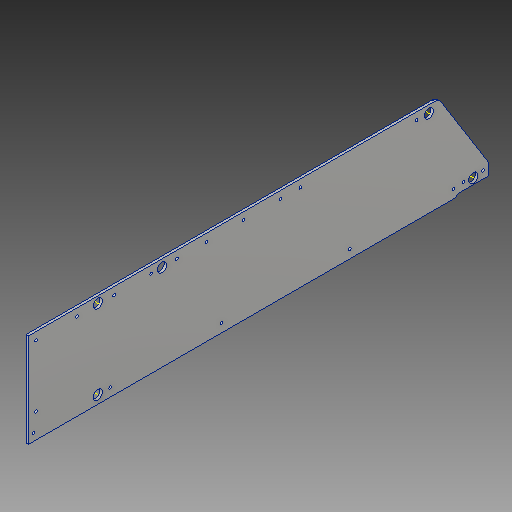
# Autodesk Inventor part: Storage Side Plate
Saved by Autodesk Inventor 2019.4 (Build 234330000, 330)
## iProperties
Created: 2020-01-24
Part Number: Storage Side Plate
Material: Aluminum 6061
Document SubType Name: Modeling
Designer: admin
Density: 2.7 g/cm^3
Appearance: Aluminum - Flat
Mass: 2248.08 g
Surface Area: 3469.21 cm^2
Volume: 832.621 cm^3
Author: admin
Autodesk Inventor part; units mm, degrees
ref_plane "YZ Plane" through (0, 0, 0) normal (1, 0, 0) x (0, 1, 0)
ref_plane "XZ Plane" through (0, 0, 0) normal (0, 1, 0) x (-1, 0, 0)
ref_plane "XY Plane" through (0, 0, 0) normal (0, 0, 1) x (1, 0, 0)
sketch "Sketch1" plane through (0, 0, 0) normal (1, 0, 0) x (0, 1, 0)
  line L0 (0, 0) -> (190, 0)
  line L1 (190, 0) -> (190, -830)
  line L2 (0, -930) -> (0, 0)
  circle A0 centre (95, -413.3735) radius 88.9 construction
  circle A1 centre (177, -140) radius 9.5
  circle A2 centre (17, -140) radius 9.5
  circle A3 centre (17, -900) radius 9.5
  circle A4 centre (175, -810) radius 9.5
  line L3 (17, -140) -> (17, -900) construction
  line L4 (234.971, -205) -> (-89.3496, -205) construction
  circle A5 centre (175, -270) radius 9.5
  line L5 (175, -270) -> (175, -810) construction
  line L6 (17, -140) -> (177, -140) construction
  circle A6 centre (97.3586, -237.1878) radius 88.9 construction
  circle A7 centre (99.6878, -594.5711) radius 88.9 construction
  circle A8 centre (95, -787.6266) radius 88.9 construction
  circle A9 centre (175, -300) radius 2.75
  circle A10 centre (175, -550) radius 2.75
  circle A11 centre (175, -785) radius 2.75
  circle A12 centre (17, -860) radius 2.75
  circle A13 centre (17, -650) radius 2.75
  circle A14 centre (17, -390) radius 2.75
  circle A15 centre (17, -165) radius 2.75
  circle A16 centre (50, -15) radius 2.75
  circle A17 centre (175, -15) radius 2.75
  line L7 (0, -930) -> (30, -930)
  line L8 (30, -930) -> (190, -830)
  dimension "d0" = 930
  dimension "d1" = 177.8
  dimension "d2" = 19
  dimension "d3" = 19
  dimension "d4" = 19
  dimension "d5" = 19
  dimension "d6" = 17
  dimension "d8" = 140
  dimension "d9" = 140
  dimension "d10" = 205
  dimension "d11" = 19
  dimension "d12" = 15
  dimension "d14" = 65
  dimension "d15" = 190
  dimension "d16" = 100
  dimension "d19" = 160
  dimension "d20" = 540
  dimension "d21" = 760
  dimension "d22" = 177.8
  dimension "d23" = 177.8
  dimension "d24" = 177.8
  dimension "d35" = 5.5
  dimension "d36" = 5.5
  dimension "d37" = 5.5
  dimension "d38" = 30
  dimension "d39" = 25
  dimension "d40" = 250
  dimension "d41" = 5.5
  dimension "d42" = 5.5
  dimension "d43" = 5.5
  dimension "d44" = 5.5
  dimension "d45" = 5.5
  dimension "d46" = 5.5
  dimension "d47" = 25
  dimension "d48" = 40
  dimension "d49" = 250
  dimension "d50" = 250
  dimension "d51" = 50
  dimension "d52" = 15
  dimension "d53" = 15
  dimension "d54" = 15
  dimension "d55" = 30
  constraints: 18 centre point, 18 end point, 7 point on line, 3 horizontal, 2 vertical, 1 parallel, 1 perpendicular
  measures "d0" distance of L2.start L0.start
  measures "d1" diameter of A0
  measures "d2" diameter of A1
  measures "d3" diameter of A2
  measures "d4" diameter of A3
  measures "d5" diameter of A4
  measures "d6" distance between parallel lines of L2 L3
  measures "d8" distance from line of L0 L6.end
  measures "d9" distance from line of L0 L3.start
  measures "d10" distance between parallel lines of L0 L4
  measures "d11" diameter of A5
  measures "d12" distance between parallel lines of L1 L5
  measures "d14" distance from line of L4 L5.start
  measures "d15" distance of L0.start L0.end
  measures "d16" vertical distance of L1.end L2.start
  measures "d19" distance of L3.start L6.end
  measures "d20" distance of L5.start L5.end
  measures "d21" distance of L3.start L3.end
  measures "d22" diameter of A6
  measures "d23" diameter of A7
  measures "d24" diameter of A8
  measures "d35" diameter of A9
  measures "d36" diameter of A10
  measures "d37" diameter of A11
  measures "d38" distance of L5.start A9.centre
  measures "d39" distance of L5.end A11.centre
  measures "d40" distance of A9.centre A10.centre
  measures "d41" diameter of A12
  measures "d42" diameter of A13
  measures "d43" diameter of A14
  measures "d44" diameter of A15
  measures "d45" diameter of A16
  measures "d46" diameter of A17
  measures "d47" distance of L3.start A15.centre
  measures "d48" distance of L3.end A12.centre
  measures "d49" distance of L3.end A13.centre
  measures "d50" distance of L3.start A14.centre
  measures "d51" distance from line of L2 A16.centre
  measures "d52" distance from line of L1 A17.centre
  measures "d53" distance from line of L0 A17.centre
  measures "d54" distance from line of L0 A16.centre
  measures "d55" distance of L2.start L7.end
extrude "Extrusion1" add sketch "Sketch1" along normal blind 5
ref_plane "Work Plane3" through (5, 17, -53740) normal (0, -0.9999989, 0.0014925) x (1, 0, 0)
ref_plane "Work Plane1" through (5, 177, -140) normal (0, -0.9999955, 0.0029851) x (-1, 0, 0)
ref_plane "Work Plane2" through (5, 17, -900) normal (0, 1, 0) x (-1, 0, 0)
ref_plane "Work Plane5" through (5, 177, -205) normal (0, 0, 1) x (-1, 0, 0)
ref_plane "Work Plane4" through (5, 177, -140) normal (0, 0, 1) x (-1, 0, 0)
fillet "Fillet1" radius 15 1 edges at (2.5, 190, -830)
sketch "Sketch2" plane through (5, 0, 0) normal (1, 0, 0) x (0, 0, -1)
  line L0 (930, 5) -> (865, 5)
  line L1 (865, 5) -> (865, 0)
  line L2 (0, 0) -> (930, 0) projected
  line L3 (930, 0) -> (930, 30) projected
  dimension "d30" = 5
  dimension "d31" = 65
  constraints: 4 end point, 2 point on line, 1 horizontal, 1 perpendicular
  measures "d30" distance of L0.end L1.end
  measures "d31" distance of L0.start L0.end
extrude "Extrusion2" cut sketch "Sketch2" against normal through all
fillet "Fillet3" radius 5 1 edges at (2.5, 5, -865)
sketch "Sketch3" plane through (5, 0, 0) normal (1, 0, 0) x (0, 0, -1)
  circle A0 centre (360, 175) radius 2.75 projected
  circle A1 centre (397.5, 175) radius 2.75 projected
  circle A2 centre (435, 175) radius 2.75 projected
  circle A3 centre (472.5, 175) radius 2.75 projected
  circle A4 centre (510, 175) radius 2.75 projected
  circle A5 centre (247.8091, 175) radius 2.75 projected
  circle A6 centre (172.8091, 175) radius 2.75 projected
  circle A7 centre (97.8091, 175) radius 2.75 projected
  circle A8 centre (920, 20) radius 2.75 projected
  circle A9 centre (880, 20) radius 2.75 projected
  circle A10 centre (10, 14.3) radius 2.75 projected
  point P0 (0, 0)
extrude "Extrusion3" cut sketch "Sketch3" against normal through all contours A0 | A2 | A4 | A5 | A6 | A7 | A8 | A9 | A10
body "Solid1"
